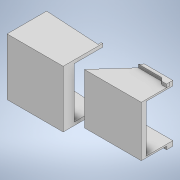
# Autodesk Inventor part: akkum
Saved by Autodesk Inventor 2020 (Build 240168000, 168)
## iProperties
Created: 2022-07-17
Part Number: akkum
Material: Типовые
Document SubType Name: Modeling
Designer: akapu
Density: 1 g/cm^3
Appearance: По умолчанию
Author: akapu
Autodesk Inventor part; units mm, degrees
ref_plane "YZ Plane" through (0, 0, 0) normal (1, 0, 0) x (0, 1, 0)
ref_plane "XZ Plane" through (0, 0, 0) normal (0, 1, 0) x (-1, 0, 0)
ref_plane "XY Plane" through (0, 0, 0) normal (0, 0, 1) x (1, 0, 0)
sketch "Эскиз1" plane through (0, 0, 0) normal (0, 1, 0) x (-1, 0, 0)
  line L0 (0, 0) -> (36, 0)
  line L1 (36, 0) -> (36, -40)
  line L2 (36, -40) -> (0, -40)
  line L3 (0, -40) -> (0, 0)
  dimension "d0" = 36
  dimension "d1" = 40
  constraints: 8 end point, 2 parallel, 1 horizontal, 1 perpendicular
  measures "d0" distance of L1.end L2.end
  measures "d1" distance of L0.end L1.end
extrude "Выдавливание1" add sketch "Эскиз1" along normal blind 1
sketch "Эскиз2" plane through (0, 1, 0) normal (0, 1, 0) x (1, 0, 0)
  line L0 (-36, 40) -> (-36, 0) projected
  line L1 (0, 0) -> (-36, 0)
  line L2 (-36, 0) -> (-36, 3)
  line L3 (-36, 3) -> (0, 3)
  line L4 (0, 3) -> (0, 0)
  dimension "d4" = 3
  constraints: 8 end point, 2 parallel, 1 horizontal, 1 perpendicular, 1 point on line
  measures "d4" distance of L1.end L2.end
extrude "Выдавливание2" add sketch "Эскиз2" along normal blind 30
sketch "Эскиз3" plane through (0, 31, 0) normal (0, 1, 0) x (1, 0, 0)
  line L0 (0, 0) -> (0, 40) projected
  line L1 (0, 0) -> (-36, 0)
  line L2 (-36, 0) -> (-36, 40)
  line L3 (-36, 40) -> (0, 40)
  line L4 (0, 40) -> (0, 0)
  constraints: 8 end point, 2 parallel, 1 horizontal, 1 perpendicular
extrude "Выдавливание3" add sketch "Эскиз3" along normal blind 1
sketch "Эскиз4" plane through (0, 32, 0) normal (0, 1, 0) x (1, 0, 0)
  line L0 (-36, 40) -> (-36, 0) projected
  line L1 (-36, 0) -> (0, 40)
  line L2 (0, 40) -> (0, 20)
  line L3 (0, 20) -> (-18, 20)
  line L4 (0, 40) -> (-36, 40) projected
  line L5 (-36, 40) -> (0, 40)
  point P0 (0, 0)
  constraints: 8 end point, 1 horizontal, 1 midpoint, 1 parallel, 1 perpendicular
extrude "Выдавливание4" cut sketch "Эскиз4" against normal blind 100
sketch "Эскиз6" plane through (0, 32, 0) normal (0, 1, 0) x (1, 0, 0)
  line L0 (0.002, 19.9819) -> (0, 17.9819)
  line L1 (0, 0) -> (0, 20) projected
  line L2 (0, 17.9819) -> (-19.7984, 18.0018)
  line L3 (-18, 20) -> (-36, 0) projected
  line L4 (-18, 20) -> (-19.7984, 18.0018)
  line L5 (-18, 20) -> (0.002, 19.9819)
  line L6 (0, 17.9819) -> (-0.002, 15.9819)
  line L7 (-0.002, 15.9819) -> (-3.002, 15.9849)
  line L8 (-3.002, 15.9849) -> (-5.3377, 17.9873)
  point P0 (0, 19.9819)
  dimension "d11" = 2
  dimension "d12" = 2
  dimension "d13" = 3
  constraints: 14 end point, 2 perpendicular, 2 point on line, 1 collinear, 1 parallel, 2 other
  measures "d11" distance of L0.start L0.end
  measures "d12" distance of L0.end L6.end
  measures "d13" distance of L6.end L7.end
extrude "Выдавливание5" add sketch "Эскиз6" along normal blind 2
sketch "Эскиз7" plane through (0, 0, 0) normal (0, -1, 0) x (1, 0, 0)
  line L0 (0, -20) -> (0, -16)
  line L1 (0, -16) -> (0, -18)
  line L2 (0, -3) -> (0, -20) projected
  line L3 (-5.3377, -17.9873) -> (-19.7984, -18.0018) projected
  line L4 (0, -18) -> (-19.7984, -18.0018)
  line L5 (-19.7984, -18.0018) -> (-18, -20)
  line L6 (-18, -20) -> (0, -20)
  line L7 (-0.002, -15.9819) -> (-3.002, -15.9849) projected
  line L8 (0, -16) -> (-3.002, -15.9849)
  line L9 (-5.3377, -17.9873) -> (-3.002, -15.9849) projected
  line L10 (-3.002, -15.9849) -> (-5.3377, -17.9873)
  point P0 (0, 0)
  dimension "d16" = 4
  dimension "d17" = 2
  constraints: 14 end point, 1 collinear, 1 point on line, 1 vertical
  measures "d16" distance of L0.start L0.end
  measures "d17" distance of L0.end L1.end
extrude "Выдавливание6" add sketch "Эскиз7" along normal blind 2 contours L6 L5 L4 L0 | L4 L3 L9 L8 L0
sketch "Эскиз8" plane through (0, 32, 0) normal (0, 1, 0) x (1, 0, 0)
  line L0 (-42.4309, 0) -> (-77.912, 0)
  line L1 (-77.912, 0) -> (-77.912, 18.0603)
  line L2 (-77.912, 18.0603) -> (-42.4309, 18.0603)
  line L3 (-42.4309, 18.0603) -> (-42.4309, 0)
  line L4 (-42.4309, 0) -> (-77.912, 0)
  line L5 (-77.912, 0) -> (-77.912, -6.9654)
  line L6 (-77.912, -6.9654) -> (-42.4309, -6.9654)
  line L7 (-42.4309, -6.9654) -> (-42.4309, 0)
  line L8 (-42.4309, 18.0603) -> (-43.4309, 18.0603)
  line L9 (-43.4309, 18.0603) -> (-43.4309, 16.0603)
  line L10 (-43.4309, 16.0603) -> (-77.912, 18.0603)
  point P0 (0, 0)
  dimension "d20" = 1
  dimension "d21" = 2
  constraints: 22 end point, 4 parallel, 3 perpendicular, 2 horizontal, 2 point on line
  measures "d20" distance of L2.end L8.end
  measures "d21" distance of L8.end L9.end
extrude "Выдавливание7" add sketch "Эскиз8" along normal blind 2 and the other way blind 34 contours L7 L6 L5 L0 | L0 L1 L10 L9 L2 L3
sketch "Эскиз9" plane through (-42.4309, -2, -18.0603) normal (1, 0, 0) x (0, 0, -1)
  line L0 (-18.0603, 34) -> (-0.0784, 34) projected
  line L1 (-0.0585, 34) -> (-18.0603, 34)
  line L2 (-18.0603, 2) -> (-2.0603, 2) projected
  line L3 (-18.0603, 34) -> (-18.0603, 2)
  line L4 (-18.0603, 2) -> (-0.0585, 2)
  line L5 (-0.0585, 2) -> (-0.0585, 34)
  line L6 (-0.0784, 34) -> (12.151, 34)
  line L7 (12.151, 34) -> (12.151, 2)
  line L8 (12.151, 2) -> (-0.0784, 2)
  line L9 (-0.0784, 2) -> (-0.0784, 34)
  point P0 (-0.0585, 34)
  constraints: 16 end point, 3 perpendicular, 2 horizontal, 2 parallel, 1 collinear
extrude "Выдавливание8" cut sketch "Эскиз9" against normal blind 40
